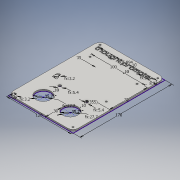
# Autodesk Inventor part: FrontPanel
Saved by Autodesk Inventor 2016 (Build 200138000, 138)
## iProperties
Created: 2015-09-18
Part Number: FrontPanel
Material: Generic
Document SubType Name: Modeling
Designer: Erin
Density: 1 g/cm^3
Appearance: Default
Author: Erin
Autodesk Inventor part; units mm, degrees
ref_plane "YZ Plane" through (0, 0, 0) normal (1, 0, 0) x (0, 1, 0)
ref_plane "XZ Plane" through (0, 0, 0) normal (0, 1, 0) x (-1, 0, 0)
ref_plane "XY Plane" through (0, 0, 0) normal (0, 0, 1) x (1, 0, 0)
sketch "Sketch1" plane through (0, 0, 0) normal (0, 0, 1) x (1, 0, 0)
  line L0 (-60, 85) -> (60, 85)
  line L1 (60, 85) -> (60, -85)
  line L2 (60, -85) -> (-60, -85)
  line L3 (-60, -85) -> (-60, 85)
  line L4 (-50, 56.6301) -> (50, 56.6301)
  line L5 (50, 56.6301) -> (50, -13.3699)
  line L6 (50, -13.3699) -> (-50, -13.3699)
  line L7 (-50, -13.3699) -> (-50, 56.6301)
  circle A0 centre (-25, -55) radius 13.85
  circle A1 centre (-25, -24.425) radius 2.7
  circle A2 centre (25, -24.425) radius 2.7
  line L8 (-25, 85) -> (-25, -85) construction
  line L9 (-60, -55) -> (60, -55) construction
  circle A3 centre (-25, -55) radius 17.875 construction
  line L10 (25, 85) -> (25, -85) construction
  circle A4 centre (25, -55) radius 13.85
  circle A5 centre (25, -55) radius 17.875 construction
  circle A6 centre (-53.4, -78.4) radius 1.6
  line L11 (-52.9471, 75) -> (52.9471, 75) construction
  line L12 (52.9471, 75) -> (52.9471, 66.6301) construction
  line L13 (52.9471, 66.6301) -> (-52.9471, 66.6301) construction
  line L14 (-52.9471, 66.6301) -> (-52.9471, 75) construction
  circle A7 centre (-43.4, -6.7699) radius 1.6
  line L15 (-50, 21.6301) -> (50, 21.6301) construction
  line L16 (0, 56.6301) -> (0, -13.3699) construction
  circle A8 centre (-43.4, 50.0301) radius 1.6
  circle A9 centre (43.4, -6.7699) radius 1.6
  circle A10 centre (43.4, 50.0301) radius 1.6
  line L17 (-60, 0) -> (60, 0) construction
  circle A11 centre (53.4, -78.4) radius 1.6
  circle A12 centre (-53.4, 78.4) radius 1.6
  circle A13 centre (53.4, 78.4) radius 1.6
  line L18 (-49.3691, 73.3171) -> (-49.3691, 72.0537)
  line L19 (-49.3691, 72.0537) -> (-50.4203, 72.0537)
  spline S0 degree 2 poles (-50.4203, 72.0537) (-50.6819, 72.0537) (-51.052, 71.6835) (-51.052, 71.422) knots 0 0 0 1 2 2 2
  line L20 (-51.052, 71.422) -> (-51.052, 70.3708)
  line L21 (-51.052, 70.3708) -> (-52.3154, 70.3708)
  line L22 (-52.3154, 70.3708) -> (-52.3154, 75)
  line L23 (-52.3154, 75) -> (-51.052, 75)
  line L24 (-51.052, 75) -> (-51.052, 73.9488)
  spline S1 degree 2 poles (-51.052, 73.9488) (-51.052, 73.6872) (-50.6819, 73.3171) (-50.4203, 73.3171) knots 0 0 0 1 2 2 2
  line L25 (-50.4203, 73.3171) -> (-49.3691, 73.3171)
  line L26 (-49.3691, 68.2634) -> (-49.3691, 67)
  line L27 (-49.3691, 67) -> (-50.4203, 67)
  spline S2 degree 2 poles (-50.4203, 67) (-50.8102, 67) (-51.506, 67.2961) (-52.0193, 67.8094) (-52.3154, 68.5052) (-52.3154, 68.8951) knots 0 0 0 1 2 3 4 4 4
  line L28 (-52.3154, 68.8951) -> (-52.3154, 69.9463)
  line L29 (-52.3154, 69.9463) -> (-51.052, 69.9463)
  line L30 (-51.052, 69.9463) -> (-51.052, 68.8951)
  spline S3 degree 2 poles (-51.052, 68.8951) (-51.052, 68.6336) (-50.6819, 68.2634) (-50.4203, 68.2634) knots 0 0 0 1 2 2 2
  line L31 (-50.4203, 68.2634) -> (-49.3691, 68.2634)
  line L32 (-45.1593, 73.3171) -> (-45.1593, 72.0537)
  line L33 (-45.1593, 72.0537) -> (-46.2105, 72.0537)
  spline S4 degree 2 poles (-46.2105, 72.0537) (-46.4721, 72.0537) (-46.8423, 71.6835) (-46.8423, 71.422) knots 0 0 0 1 2 2 2
  line L34 (-46.8423, 71.422) -> (-46.8423, 70.3708)
  line L35 (-46.8423, 70.3708) -> (-48.1057, 70.3708)
  line L36 (-48.1057, 70.3708) -> (-48.1057, 75)
  line L37 (-48.1057, 75) -> (-46.8423, 75)
  line L38 (-46.8423, 75) -> (-46.8423, 73.9488)
  spline S5 degree 2 poles (-46.8423, 73.9488) (-46.8423, 73.6872) (-46.4721, 73.3171) (-46.2105, 73.3171) knots 0 0 0 1 2 2 2
  line L39 (-46.2105, 73.3171) -> (-45.1593, 73.3171)
  line L40 (-44.7349, 72.0537) -> (-44.7349, 73.3171)
  line L41 (-44.7349, 73.3171) -> (-43.6837, 73.3171)
  spline S6 degree 2 poles (-43.6837, 73.3171) (-43.2938, 73.3171) (-42.598, 73.021) (-42.0847, 72.5077) (-41.7886, 71.8118) (-41.7886, 71.422) knots 0 0 0 1 2 3 4 4 4
  line L42 (-41.7886, 71.422) -> (-41.7886, 70.3708)
  line L43 (-41.7886, 70.3708) -> (-43.052, 70.3708)
  line L44 (-43.052, 70.3708) -> (-43.052, 71.422)
  spline S7 degree 2 poles (-43.052, 71.422) (-43.052, 71.6835) (-43.4123, 72.0537) (-43.6837, 72.0537) knots 0 0 0 1 2 2 2
  line L45 (-43.6837, 72.0537) -> (-44.7349, 72.0537)
  line L46 (-41.7886, 67) -> (-43.052, 67)
  line L47 (-43.052, 67) -> (-43.052, 69.9463)
  line L48 (-43.052, 69.9463) -> (-41.7886, 69.9463)
  line L49 (-41.7886, 69.9463) -> (-41.7886, 67)
  line L50 (-46.8423, 67) -> (-48.1057, 67)
  line L51 (-48.1057, 67) -> (-48.1057, 69.9463)
  line L52 (-48.1057, 69.9463) -> (-46.8423, 69.9463)
  line L53 (-46.8423, 69.9463) -> (-46.8423, 67)
  line L54 (-39.2617, 70.3708) -> (-40.5252, 70.3708)
  line L55 (-40.5252, 70.3708) -> (-40.5252, 71.422)
  spline S8 degree 2 poles (-40.5252, 71.422) (-40.5252, 71.8118) (-40.229, 72.5077) (-39.7158, 73.021) (-39.0199, 73.3171) (-38.63, 73.3171) knots 0 0 0 1 2 3 4 4 4
  line L56 (-38.63, 73.3171) -> (-37.5788, 73.3171)
  line L57 (-37.5788, 73.3171) -> (-37.5788, 72.0537)
  line L58 (-37.5788, 72.0537) -> (-38.63, 72.0537)
  spline S9 degree 2 poles (-38.63, 72.0537) (-38.8916, 72.0537) (-39.2617, 71.6835) (-39.2617, 71.422) knots 0 0 0 1 2 2 2
  line L59 (-39.2617, 71.422) -> (-39.2617, 70.3708)
  line L60 (-37.5788, 68.2634) -> (-37.5788, 67)
  line L61 (-37.5788, 67) -> (-38.63, 67)
  spline S10 degree 2 poles (-38.63, 67) (-39.0199, 67) (-39.7158, 67.2961) (-40.229, 67.8094) (-40.5252, 68.5052) (-40.5252, 68.8951) knots 0 0 0 1 2 3 4 4 4
  line L62 (-40.5252, 68.8951) -> (-40.5252, 69.9463)
  line L63 (-40.5252, 69.9463) -> (-39.2617, 69.9463)
  line L64 (-39.2617, 69.9463) -> (-39.2617, 68.8951)
  spline S11 degree 2 poles (-39.2617, 68.8951) (-39.2617, 68.6336) (-38.8916, 68.2634) (-38.63, 68.2634) knots 0 0 0 1 2 2 2
  line L65 (-38.63, 68.2634) -> (-37.5788, 68.2634)
  line L66 (-35.4715, 69.9463) -> (-34.2081, 69.9463)
  line L67 (-34.2081, 69.9463) -> (-34.2081, 68.8951)
  spline S12 degree 2 poles (-34.2081, 68.8951) (-34.2081, 68.5052) (-34.5042, 67.8094) (-35.0175, 67.2961) (-35.7133, 67) (-36.1032, 67) knots 0 0 0 1 2 3 4 4 4
  line L68 (-36.1032, 67) -> (-37.1544, 67)
  line L69 (-37.1544, 67) -> (-37.1544, 68.2634)
  line L70 (-37.1544, 68.2634) -> (-36.1032, 68.2634)
  spline S13 degree 2 poles (-36.1032, 68.2634) (-35.8318, 68.2634) (-35.4715, 68.6336) (-35.4715, 68.8951) knots 0 0 0 1 2 2 2
  line L71 (-35.4715, 68.8951) -> (-35.4715, 69.9463)
  line L72 (-37.1544, 72.0537) -> (-37.1544, 73.3171)
  line L73 (-37.1544, 73.3171) -> (-36.1032, 73.3171)
  spline S14 degree 2 poles (-36.1032, 73.3171) (-35.7133, 73.3171) (-35.0175, 73.021) (-34.5042, 72.5077) (-34.2081, 71.8118) (-34.2081, 71.422) knots 0 0 0 1 2 3 4 4 4
  line L74 (-34.2081, 71.422) -> (-34.2081, 70.3708)
  line L75 (-34.2081, 70.3708) -> (-35.4715, 70.3708)
  line L76 (-35.4715, 70.3708) -> (-35.4715, 71.422)
  spline S15 degree 2 poles (-35.4715, 71.422) (-35.4715, 71.6835) (-35.8318, 72.0537) (-36.1032, 72.0537) knots 0 0 0 1 2 2 2
  line L77 (-36.1032, 72.0537) -> (-37.1544, 72.0537)
  spline S16 degree 2 poles (-27.891, 68.8951) (-27.891, 68.6336) (-28.2513, 68.2634) (-28.5227, 68.2634) knots 0 0 0 1 2 2 2
  line L78 (-28.5227, 68.2634) -> (-29.5788, 68.2634)
  line L79 (-29.5788, 68.2634) -> (-29.5788, 67)
  line L80 (-29.5788, 67) -> (-28.5227, 67)
  spline S17 degree 2 poles (-28.5227, 67) (-28.1328, 67) (-27.4369, 67.2961) (-26.9237, 67.8094) (-26.6276, 68.5052) (-26.6276, 68.8951) knots 0 0 0 1 2 3 4 4 4
  line L81 (-26.6276, 68.8951) -> (-26.6276, 69.9463)
  line L82 (-26.6276, 69.9463) -> (-27.891, 69.9463)
  line L83 (-27.891, 69.9463) -> (-27.891, 68.8951)
  spline S18 degree 2 poles (-31.0495, 68.2634) (-31.3111, 68.2634) (-31.6812, 68.6336) (-31.6812, 68.8951) knots 0 0 0 1 2 2 2
  line L84 (-31.6812, 68.8951) -> (-31.6812, 69.9463)
  line L85 (-31.6812, 69.9463) -> (-32.9447, 69.9463)
  line L86 (-32.9447, 69.9463) -> (-32.9447, 68.8951)
  spline S19 degree 2 poles (-32.9447, 68.8951) (-32.9447, 68.5052) (-32.6485, 67.8094) (-32.1353, 67.2961) (-31.4394, 67) (-31.0495, 67) knots 0 0 0 1 2 3 4 4 4
  line L87 (-31.0495, 67) -> (-29.9983, 67)
  line L88 (-29.9983, 67) -> (-29.9983, 68.2634)
  line L89 (-29.9983, 68.2634) -> (-31.0495, 68.2634)
  line L90 (-32.9447, 73.3171) -> (-31.6812, 73.3171)
  line L91 (-31.6812, 73.3171) -> (-31.6812, 70.3708)
  line L92 (-31.6812, 70.3708) -> (-32.9447, 70.3708)
  line L93 (-32.9447, 70.3708) -> (-32.9447, 73.3171)
  line L94 (-27.891, 73.3171) -> (-26.6276, 73.3171)
  line L95 (-26.6276, 73.3171) -> (-26.6276, 70.3708)
  line L96 (-26.6276, 70.3708) -> (-27.891, 70.3708)
  line L97 (-27.891, 70.3708) -> (-27.891, 73.3171)
  line L98 (-20.73, 68.2634) -> (-20.73, 67)
  line L99 (-20.73, 67) -> (-23.469, 67)
  spline S20 degree 2 poles (-23.469, 67) (-23.8589, 67) (-24.5548, 67.2961) (-25.068, 67.8094) (-25.3641, 68.5052) (-25.3641, 68.8951) knots 0 0 0 1 2 3 4 4 4
  line L100 (-25.3641, 68.8951) -> (-25.3641, 69.9463)
  line L101 (-25.3641, 69.9463) -> (-24.1007, 69.9463)
  line L102 (-24.1007, 69.9463) -> (-24.1007, 68.8951)
  spline S21 degree 2 poles (-24.1007, 68.8951) (-24.1007, 68.6336) (-23.7306, 68.2634) (-23.469, 68.2634) knots 0 0 0 1 2 2 2
  line L103 (-23.469, 68.2634) -> (-20.73, 68.2634)
  line L104 (-20.3105, 69.9513) -> (-19.0471, 69.9513)
  line L105 (-19.0471, 69.9513) -> (-19.0471, 67.2122)
  spline S22 degree 2 poles (-19.0471, 67.2122) (-19.0471, 66.8223) (-19.3432, 66.1265) (-19.8564, 65.6132) (-20.5523, 65.3171) (-20.9422, 65.3171) knots 0 0 0 1 2 3 4 4 4
  line L106 (-20.9422, 65.3171) -> (-21.9934, 65.3171)
  line L107 (-21.9934, 65.3171) -> (-21.9934, 66.5805)
  line L108 (-21.9934, 66.5805) -> (-20.9422, 66.5805)
  spline S23 degree 2 poles (-20.9422, 66.5805) (-20.6708, 66.5805) (-20.3105, 66.9506) (-20.3105, 67.2122) knots 0 0 0 1 2 2 2
  line L109 (-20.3105, 67.2122) -> (-20.3105, 69.9513)
  line L110 (-24.1007, 70.3708) -> (-25.3641, 70.3708)
  line L111 (-25.3641, 70.3708) -> (-25.3641, 71.422)
  spline S24 degree 2 poles (-25.3641, 71.422) (-25.3641, 71.8118) (-25.068, 72.5077) (-24.5548, 73.021) (-23.8589, 73.3171) (-23.469, 73.3171) knots 0 0 0 1 2 3 4 4 4
  line L112 (-23.469, 73.3171) -> (-22.4178, 73.3171)
  line L113 (-22.4178, 73.3171) -> (-22.4178, 72.0537)
  line L114 (-22.4178, 72.0537) -> (-23.469, 72.0537)
  spline S25 degree 2 poles (-23.469, 72.0537) (-23.7306, 72.0537) (-24.1007, 71.6835) (-24.1007, 71.422) knots 0 0 0 1 2 2 2
  line L115 (-24.1007, 71.422) -> (-24.1007, 70.3708)
  line L116 (-21.9934, 72.0537) -> (-21.9934, 73.3171)
  line L117 (-21.9934, 73.3171) -> (-20.9422, 73.3171)
  spline S26 degree 2 poles (-20.9422, 73.3171) (-20.5523, 73.3171) (-19.8564, 73.021) (-19.3432, 72.5077) (-19.0471, 71.8118) (-19.0471, 71.422) knots 0 0 0 1 2 3 4 4 4
  line L118 (-19.0471, 71.422) -> (-19.0471, 70.3708)
  line L119 (-19.0471, 70.3708) -> (-20.3105, 70.3708)
  line L120 (-20.3105, 70.3708) -> (-20.3105, 71.422)
  spline S27 degree 2 poles (-20.3105, 71.422) (-20.3105, 71.6835) (-20.6708, 72.0537) (-20.9422, 72.0537) knots 0 0 0 1 2 2 2
  line L121 (-20.9422, 72.0537) -> (-21.9934, 72.0537)
  line L122 (-22.4178, 66.5805) -> (-22.4178, 65.3171)
  line L123 (-22.4178, 65.3171) -> (-25.3641, 65.3171)
  line L124 (-25.3641, 65.3171) -> (-25.3641, 66.5805)
  line L125 (-25.3641, 66.5805) -> (-22.4178, 66.5805)
  line L126 (-14.8373, 73.3171) -> (-14.8373, 72.0537)
  line L127 (-14.8373, 72.0537) -> (-15.8885, 72.0537)
  spline S28 degree 2 poles (-15.8885, 72.0537) (-16.1501, 72.0537) (-16.5202, 71.6835) (-16.5202, 71.422) knots 0 0 0 1 2 2 2
  line L128 (-16.5202, 71.422) -> (-16.5202, 70.3708)
  line L129 (-16.5202, 70.3708) -> (-17.7836, 70.3708)
  line L130 (-17.7836, 70.3708) -> (-17.7836, 75)
  line L131 (-17.7836, 75) -> (-16.5202, 75)
  line L132 (-16.5202, 75) -> (-16.5202, 73.9488)
  spline S29 degree 2 poles (-16.5202, 73.9488) (-16.5202, 73.6872) (-16.1501, 73.3171) (-15.8885, 73.3171) knots 0 0 0 1 2 2 2
  line L133 (-15.8885, 73.3171) -> (-14.8373, 73.3171)
  line L134 (-14.4129, 72.0537) -> (-14.4129, 73.3171)
  line L135 (-14.4129, 73.3171) -> (-13.3617, 73.3171)
  spline S30 degree 2 poles (-13.3617, 73.3171) (-12.9718, 73.3171) (-12.2759, 73.021) (-11.7627, 72.5077) (-11.4666, 71.8118) (-11.4666, 71.422) knots 0 0 0 1 2 3 4 4 4
  line L136 (-11.4666, 71.422) -> (-11.4666, 70.3708)
  line L137 (-11.4666, 70.3708) -> (-12.73, 70.3708)
  line L138 (-12.73, 70.3708) -> (-12.73, 71.422)
  spline S31 degree 2 poles (-12.73, 71.422) (-12.73, 71.6835) (-13.0902, 72.0537) (-13.3617, 72.0537) knots 0 0 0 1 2 2 2
  line L139 (-13.3617, 72.0537) -> (-14.4129, 72.0537)
  line L140 (-11.4666, 67) -> (-12.73, 67)
  line L141 (-12.73, 67) -> (-12.73, 69.9463)
  line L142 (-12.73, 69.9463) -> (-11.4666, 69.9463)
  line L143 (-11.4666, 69.9463) -> (-11.4666, 67)
  line L144 (-16.5202, 67) -> (-17.7836, 67)
  line L145 (-17.7836, 67) -> (-17.7836, 69.9463)
  line L146 (-17.7836, 69.9463) -> (-16.5202, 69.9463)
  line L147 (-16.5202, 69.9463) -> (-16.5202, 67)
  line L148 (-7.2568, 73.3171) -> (-7.2568, 72.0537)
  line L149 (-7.2568, 72.0537) -> (-8.308, 72.0537)
  spline S32 degree 2 poles (-8.308, 72.0537) (-8.5696, 72.0537) (-8.9397, 71.6835) (-8.9397, 71.422) knots 0 0 0 1 2 2 2
  line L150 (-8.9397, 71.422) -> (-8.9397, 70.3708)
  line L151 (-8.9397, 70.3708) -> (-10.2031, 70.3708)
  line L152 (-10.2031, 70.3708) -> (-10.2031, 75)
  line L153 (-10.2031, 75) -> (-8.9397, 75)
  line L154 (-8.9397, 75) -> (-8.9397, 73.9488)
  spline S33 degree 2 poles (-8.9397, 73.9488) (-8.9397, 73.6872) (-8.5696, 73.3171) (-8.308, 73.3171) knots 0 0 0 1 2 2 2
  line L155 (-8.308, 73.3171) -> (-7.2568, 73.3171)
  line L156 (-7.2568, 68.2634) -> (-7.2568, 67)
  line L157 (-7.2568, 67) -> (-8.308, 67)
  spline S34 degree 2 poles (-8.308, 67) (-8.6979, 67) (-9.3938, 67.2961) (-9.907, 67.8094) (-10.2031, 68.5052) (-10.2031, 68.8951) knots 0 0 0 1 2 3 4 4 4
  line L158 (-10.2031, 68.8951) -> (-10.2031, 69.9463)
  line L159 (-10.2031, 69.9463) -> (-8.9397, 69.9463)
  line L160 (-8.9397, 69.9463) -> (-8.9397, 68.8951)
  spline S35 degree 2 poles (-8.9397, 68.8951) (-8.9397, 68.6336) (-8.5696, 68.2634) (-8.308, 68.2634) knots 0 0 0 1 2 2 2
  line L161 (-8.308, 68.2634) -> (-7.2568, 68.2634)
  spline S36 degree 2 poles (-1.1519, 67) (-1.4135, 67) (-1.7836, 66.6299) (-1.7836, 66.3683) knots 0 0 0 1 2 2 2
  line L162 (-1.7836, 66.3683) -> (-1.7836, 65.3171)
  line L163 (-1.7836, 65.3171) -> (-3.0471, 65.3171)
  line L164 (-3.0471, 65.3171) -> (-3.0471, 69.9463)
  line L165 (-3.0471, 69.9463) -> (-1.7836, 69.9463)
  line L166 (-1.7836, 69.9463) -> (-1.7836, 68.8951)
  spline S37 degree 2 poles (-1.7836, 68.8951) (-1.7836, 68.6336) (-1.4135, 68.2634) (-1.1519, 68.2634) knots 0 0 0 1 2 2 2
  line L167 (-1.1519, 68.2634) -> (-0.1007, 68.2634)
  line L168 (-0.1007, 68.2634) -> (-0.1007, 67)
  line L169 (-0.1007, 67) -> (-1.1519, 67)
  spline S38 degree 2 poles (-1.1519, 72.0537) (-1.4135, 72.0537) (-1.7836, 71.6835) (-1.7836, 71.422) knots 0 0 0 1 2 2 2
  line L170 (-1.7836, 71.422) -> (-1.7836, 70.3708)
  line L171 (-1.7836, 70.3708) -> (-3.0471, 70.3708)
  line L172 (-3.0471, 70.3708) -> (-3.0471, 71.422)
  spline S39 degree 2 poles (-3.0471, 71.422) (-3.0471, 71.8118) (-2.7509, 72.5077) (-2.2377, 73.021) (-1.5418, 73.3171) (-1.1519, 73.3171) knots 0 0 0 1 2 3 4 4 4
  line L173 (-1.1519, 73.3171) -> (-0.1007, 73.3171)
  line L174 (-0.1007, 73.3171) -> (-0.1007, 72.0537)
  line L175 (-0.1007, 72.0537) -> (-1.1519, 72.0537)
  spline S40 degree 2 poles (2.0066, 71.422) (2.0066, 71.6835) (1.6463, 72.0537) (1.3749, 72.0537) knots 0 0 0 1 2 2 2
  line L176 (1.3749, 72.0537) -> (0.3237, 72.0537)
  line L177 (0.3237, 72.0537) -> (0.3237, 73.3171)
  line L178 (0.3237, 73.3171) -> (1.3749, 73.3171)
  spline S41 degree 2 poles (1.3749, 73.3171) (1.7648, 73.3171) (2.4607, 73.021) (2.9739, 72.5077) (3.27, 71.8118) (3.27, 71.422) knots 0 0 0 1 2 3 4 4 4
  line L179 (3.27, 71.422) -> (3.27, 70.3708)
  line L180 (3.27, 70.3708) -> (2.0066, 70.3708)
  line L181 (2.0066, 70.3708) -> (2.0066, 71.422)
  spline S42 degree 2 poles (1.3749, 68.2634) (1.6463, 68.2634) (2.0066, 68.6336) (2.0066, 68.8951) knots 0 0 0 1 2 2 2
  line L182 (2.0066, 68.8951) -> (2.0066, 69.9463)
  line L183 (2.0066, 69.9463) -> (3.27, 69.9463)
  line L184 (3.27, 69.9463) -> (3.27, 68.8951)
  spline S43 degree 2 poles (3.27, 68.8951) (3.27, 68.5052) (2.9739, 67.8094) (2.4607, 67.2961) (1.7648, 67) (1.3749, 67) knots 0 0 0 1 2 3 4 4 4
  line L185 (1.3749, 67) -> (0.3237, 67)
  line L186 (0.3237, 67) -> (0.3237, 68.2634)
  line L187 (0.3237, 68.2634) -> (1.3749, 68.2634)
  spline S44 degree 2 poles (6.4286, 72.0537) (6.167, 72.0537) (5.7969, 71.6835) (5.7969, 71.422) knots 0 0 0 1 2 2 2
  line L188 (5.7969, 71.422) -> (5.7969, 70.3708)
  line L189 (5.7969, 70.3708) -> (4.5334, 70.3708)
  line L190 (4.5334, 70.3708) -> (4.5334, 71.422)
  spline S45 degree 2 poles (4.5334, 71.422) (4.5334, 71.8118) (4.8296, 72.5077) (5.3428, 73.021) (6.0387, 73.3171) (6.4286, 73.3171) knots 0 0 0 1 2 3 4 4 4
  line L191 (6.4286, 73.3171) -> (9.1676, 73.3171)
  line L192 (9.1676, 73.3171) -> (9.1676, 72.0537)
  line L193 (9.1676, 72.0537) -> (6.4286, 72.0537)
  line L194 (5.7969, 67) -> (4.5334, 67)
  line L195 (4.5334, 67) -> (4.5334, 69.9463)
  line L196 (4.5334, 69.9463) -> (5.7969, 69.9463)
  line L197 (5.7969, 69.9463) -> (5.7969, 67)
  line L198 (11.6895, 70.3708) -> (10.4261, 70.3708)
  line L199 (10.4261, 70.3708) -> (10.4261, 71.422)
  spline S46 degree 2 poles (10.4261, 71.422) (10.4261, 71.8118) (10.7222, 72.5077) (11.2355, 73.021) (11.9313, 73.3171) (12.3212, 73.3171) knots 0 0 0 1 2 3 4 4 4
  line L200 (12.3212, 73.3171) -> (13.3724, 73.3171)
  line L201 (13.3724, 73.3171) -> (13.3724, 72.0537)
  line L202 (13.3724, 72.0537) -> (12.3212, 72.0537)
  spline S47 degree 2 poles (12.3212, 72.0537) (12.0597, 72.0537) (11.6895, 71.6835) (11.6895, 71.422) knots 0 0 0 1 2 2 2
  line L203 (11.6895, 71.422) -> (11.6895, 70.3708)
  line L204 (13.3724, 68.2634) -> (13.3724, 67)
  line L205 (13.3724, 67) -> (12.3212, 67)
  spline S48 degree 2 poles (12.3212, 67) (11.9313, 67) (11.2355, 67.2961) (10.7222, 67.8094) (10.4261, 68.5052) (10.4261, 68.8951) knots 0 0 0 1 2 3 4 4 4
  line L206 (10.4261, 68.8951) -> (10.4261, 69.9463)
  line L207 (10.4261, 69.9463) -> (11.6895, 69.9463)
  line L208 (11.6895, 69.9463) -> (11.6895, 68.8951)
  spline S49 degree 2 poles (11.6895, 68.8951) (11.6895, 68.6336) (12.0597, 68.2634) (12.3212, 68.2634) knots 0 0 0 1 2 2 2
  line L209 (12.3212, 68.2634) -> (13.3724, 68.2634)
  line L210 (13.7969, 72.0537) -> (13.7969, 73.3171)
  line L211 (13.7969, 73.3171) -> (14.8481, 73.3171)
  spline S50 degree 2 poles (14.8481, 73.3171) (15.2379, 73.3171) (15.9338, 73.021) (16.4471, 72.5077) (16.7432, 71.8118) (16.7432, 71.422) knots 0 0 0 1 2 3 4 4 4
  line L212 (16.7432, 71.422) -> (16.7432, 70.3708)
  line L213 (16.7432, 70.3708) -> (15.4798, 70.3708)
  line L214 (15.4798, 70.3708) -> (15.4798, 71.422)
  spline S51 degree 2 poles (15.4798, 71.422) (15.4798, 71.6835) (15.1195, 72.0537) (14.8481, 72.0537) knots 0 0 0 1 2 2 2
  line L215 (14.8481, 72.0537) -> (13.7969, 72.0537)
  line L216 (15.4798, 69.9463) -> (16.7432, 69.9463)
  line L217 (16.7432, 69.9463) -> (16.7432, 68.8951)
  spline S52 degree 2 poles (16.7432, 68.8951) (16.7432, 68.5052) (16.4471, 67.8094) (15.9338, 67.2961) (15.2379, 67) (14.8481, 67) knots 0 0 0 1 2 3 4 4 4
  line L218 (14.8481, 67) -> (13.7969, 67)
  line L219 (13.7969, 67) -> (13.7969, 68.2634)
  line L220 (13.7969, 68.2634) -> (14.8481, 68.2634)
  spline S53 degree 2 poles (14.8481, 68.2634) (15.1195, 68.2634) (15.4798, 68.6336) (15.4798, 68.8951) knots 0 0 0 1 2 2 2
  line L221 (15.4798, 68.8951) -> (15.4798, 69.9463)
  spline S54 degree 2 poles (20.7457, 72.0537) (21.0171, 72.0537) (21.3774, 71.6835) (21.3774, 71.422) knots 0 0 0 1 2 2 2
  line L222 (21.3774, 71.422) -> (21.3774, 70.3708)
  line L223 (21.3774, 70.3708) -> (22.6408, 70.3708)
  line L224 (22.6408, 70.3708) -> (22.6408, 71.422)
  spline S55 degree 2 poles (22.6408, 71.422) (22.6408, 71.8118) (22.3447, 72.5077) (21.8314, 73.021) (21.1355, 73.3171) (20.7457, 73.3171) knots 0 0 0 1 2 3 4 4 4
  line L225 (20.7457, 73.3171) -> (19.6945, 73.3171)
  line L226 (19.6945, 73.3171) -> (19.6945, 72.0537)
  line L227 (19.6945, 72.0537) -> (20.7457, 72.0537)
  spline S56 degree 2 poles (24.1115, 72.0537) (24.3879, 72.0537) (24.7432, 71.6835) (24.7432, 71.422) knots 0 0 0 1 2 2 2
  line L228 (24.7432, 71.422) -> (24.7432, 70.3708)
  line L229 (24.7432, 70.3708) -> (26.0066, 70.3708)
  line L230 (26.0066, 70.3708) -> (26.0066, 71.422)
  spline S57 degree 2 poles (26.0066, 71.422) (26.0066, 71.8118) (25.7105, 72.5077) (25.1972, 73.021) (24.5014, 73.3171) (24.1115, 73.3171) knots 0 0 0 1 2 3 4 4 4
  line L231 (24.1115, 73.3171) -> (23.0603, 73.3171)
  line L232 (23.0603, 73.3171) -> (23.0603, 72.0537)
  line L233 (23.0603, 72.0537) -> (24.1115, 72.0537)
  line L234 (26.0066, 67) -> (24.7432, 67)
  line L235 (24.7432, 67) -> (24.7432, 69.9463)
  line L236 (24.7432, 69.9463) -> (26.0066, 69.9463)
  line L237 (26.0066, 69.9463) -> (26.0066, 67)
  line L238 (22.6408, 67) -> (21.3774, 67)
  line L239 (21.3774, 67) -> (21.3774, 69.9463)
  line L240 (21.3774, 69.9463) -> (22.6408, 69.9463)
  line L241 (22.6408, 69.9463) -> (22.6408, 67)
  line L242 (19.27, 70.3708) -> (18.0066, 70.3708)
  line L243 (18.0066, 70.3708) -> (18.0066, 73.3171)
  line L244 (18.0066, 73.3171) -> (19.27, 73.3171)
  line L245 (19.27, 73.3171) -> (19.27, 70.3708)
  line L246 (19.27, 67) -> (18.0066, 67)
  line L247 (18.0066, 67) -> (18.0066, 69.9463)
  line L248 (18.0066, 69.9463) -> (19.27, 69.9463)
  line L249 (19.27, 69.9463) -> (19.27, 67)
  spline S58 degree 2 poles (29.1652, 67) (28.9036, 67) (28.5334, 66.6299) (28.5334, 66.3683) knots 0 0 0 1 2 2 2
  line L250 (28.5334, 66.3683) -> (28.5334, 65.3171)
  line L251 (28.5334, 65.3171) -> (27.27, 65.3171)
  line L252 (27.27, 65.3171) -> (27.27, 69.9463)
  line L253 (27.27, 69.9463) -> (28.5334, 69.9463)
  line L254 (28.5334, 69.9463) -> (28.5334, 68.8951)
  spline S59 degree 2 poles (28.5334, 68.8951) (28.5334, 68.6336) (28.9036, 68.2634) (29.1652, 68.2634) knots 0 0 0 1 2 2 2
  line L255 (29.1652, 68.2634) -> (30.2164, 68.2634)
  line L256 (30.2164, 68.2634) -> (30.2164, 67)
  line L257 (30.2164, 67) -> (29.1652, 67)
  spline S60 degree 2 poles (29.1652, 72.0537) (28.9036, 72.0537) (28.5334, 71.6835) (28.5334, 71.422) knots 0 0 0 1 2 2 2
  line L258 (28.5334, 71.422) -> (28.5334, 70.3708)
  line L259 (28.5334, 70.3708) -> (27.27, 70.3708)
  line L260 (27.27, 70.3708) -> (27.27, 71.422)
  spline S61 degree 2 poles (27.27, 71.422) (27.27, 71.8118) (27.5661, 72.5077) (28.0794, 73.021) (28.7753, 73.3171) (29.1652, 73.3171) knots 0 0 0 1 2 3 4 4 4
  line L261 (29.1652, 73.3171) -> (30.2164, 73.3171)
  line L262 (30.2164, 73.3171) -> (30.2164, 72.0537)
  line L263 (30.2164, 72.0537) -> (29.1652, 72.0537)
  spline S62 degree 2 poles (32.3237, 71.422) (32.3237, 71.6835) (31.9634, 72.0537) (31.692, 72.0537) knots 0 0 0 1 2 2 2
  line L264 (31.692, 72.0537) -> (30.6408, 72.0537)
  line L265 (30.6408, 72.0537) -> (30.6408, 73.3171)
  line L266 (30.6408, 73.3171) -> (31.692, 73.3171)
  spline S63 degree 2 poles (31.692, 73.3171) (32.0819, 73.3171) (32.7777, 73.021) (33.291, 72.5077) (33.5871, 71.8118) (33.5871, 71.422) knots 0 0 0 1 2 3 4 4 4
  line L267 (33.5871, 71.422) -> (33.5871, 70.3708)
  line L268 (33.5871, 70.3708) -> (32.3237, 70.3708)
  line L269 (32.3237, 70.3708) -> (32.3237, 71.422)
  spline S64 degree 2 poles (31.692, 68.2634) (31.9634, 68.2634) (32.3237, 68.6336) (32.3237, 68.8951) knots 0 0 0 1 2 2 2
  line L270 (32.3237, 68.8951) -> (32.3237, 69.9463)
  line L271 (32.3237, 69.9463) -> (33.5871, 69.9463)
  line L272 (33.5871, 69.9463) -> (33.5871, 68.8951)
  spline S65 degree 2 poles (33.5871, 68.8951) (33.5871, 68.5052) (33.291, 67.8094) (32.7777, 67.2961) (32.0819, 67) (31.692, 67) knots 0 0 0 1 2 3 4 4 4
  line L273 (31.692, 67) -> (30.6408, 67)
  line L274 (30.6408, 67) -> (30.6408, 68.2634)
  line L275 (30.6408, 68.2634) -> (31.692, 68.2634)
  line L276 (37.7969, 73.3171) -> (37.7969, 72.0537)
  line L277 (37.7969, 72.0537) -> (36.7457, 72.0537)
  spline S66 degree 2 poles (36.7457, 72.0537) (36.4841, 72.0537) (36.114, 71.6835) (36.114, 71.422) knots 0 0 0 1 2 2 2
  line L278 (36.114, 71.422) -> (36.114, 70.3708)
  line L279 (36.114, 70.3708) -> (34.8505, 70.3708)
  line L280 (34.8505, 70.3708) -> (34.8505, 75)
  line L281 (34.8505, 75) -> (36.114, 75)
  line L282 (36.114, 75) -> (36.114, 73.9488)
  spline S67 degree 2 poles (36.114, 73.9488) (36.114, 73.6872) (36.4841, 73.3171) (36.7457, 73.3171) knots 0 0 0 1 2 2 2
  line L283 (36.7457, 73.3171) -> (37.7969, 73.3171)
  line L284 (37.7969, 68.2634) -> (37.7969, 67)
  line L285 (37.7969, 67) -> (36.7457, 67)
  spline S68 degree 2 poles (36.7457, 67) (36.3558, 67) (35.6599, 67.2961) (35.1466, 67.8094) (34.8505, 68.5052) (34.8505, 68.8951) knots 0 0 0 1 2 3 4 4 4
  line L286 (34.8505, 68.8951) -> (34.8505, 69.9463)
  line L287 (34.8505, 69.9463) -> (36.114, 69.9463)
  line L288 (36.114, 69.9463) -> (36.114, 68.8951)
  spline S69 degree 2 poles (36.114, 68.8951) (36.114, 68.6336) (36.4841, 68.2634) (36.7457, 68.2634) knots 0 0 0 1 2 2 2
  line L289 (36.7457, 68.2634) -> (37.7969, 68.2634)
  spline S70 degree 2 poles (44.114, 71.422) (44.114, 71.6835) (43.7537, 72.0537) (43.4822, 72.0537) knots 0 0 0 1 2 2 2
  line L290 (43.4822, 72.0537) -> (42.431, 72.0537)
  line L291 (42.431, 72.0537) -> (42.431, 73.3171)
  line L292 (42.431, 73.3171) -> (43.4822, 73.3171)
  spline S71 degree 2 poles (43.4822, 73.3171) (43.8721, 73.3171) (44.568, 73.021) (45.0813, 72.5077) (45.3774, 71.8118) (45.3774, 71.422) knots 0 0 0 1 2 3 4 4 4
  line L293 (45.3774, 71.422) -> (45.3774, 70.578)
  spline S72 degree 2 poles (45.3774, 70.578) (45.3774, 70.1882) (45.0813, 69.4923) (44.568, 68.979) (43.8721, 68.6829) (43.4822, 68.6829) knots 0 0 0 1 2 3 4 4 4
  line L294 (43.4822, 68.6829) -> (42.431, 68.6829)
  line L295 (42.431, 68.6829) -> (42.431, 69.9463)
  line L296 (42.431, 69.9463) -> (43.4822, 69.9463)
  spline S73 degree 2 poles (43.4822, 69.9463) (43.7537, 69.9463) (44.114, 70.3165) (44.114, 70.578) knots 0 0 0 1 2 2 2
  line L297 (44.114, 70.578) -> (44.114, 71.422)
  line L298 (40.3237, 70.3708) -> (39.0603, 70.3708)
  line L299 (39.0603, 70.3708) -> (39.0603, 71.422)
  spline S74 degree 2 poles (39.0603, 71.422) (39.0603, 71.8118) (39.3564, 72.5077) (39.8697, 73.021) (40.5655, 73.3171) (40.9554, 73.3171) knots 0 0 0 1 2 3 4 4 4
  line L300 (40.9554, 73.3171) -> (42.0066, 73.3171)
  line L301 (42.0066, 73.3171) -> (42.0066, 72.0537)
  line L302 (42.0066, 72.0537) -> (40.9554, 72.0537)
  spline S75 degree 2 poles (40.9554, 72.0537) (40.6938, 72.0537) (40.3237, 71.6835) (40.3237, 71.422) knots 0 0 0 1 2 2 2
  line L303 (40.3237, 71.422) -> (40.3237, 70.3708)
  line L304 (42.0066, 68.2634) -> (42.0066, 67)
  line L305 (42.0066, 67) -> (40.9554, 67)
  spline S76 degree 2 poles (40.9554, 67) (40.5655, 67) (39.8697, 67.2961) (39.3564, 67.8094) (39.0603, 68.5052) (39.0603, 68.8951) knots 0 0 0 1 2 3 4 4 4
  line L306 (39.0603, 68.8951) -> (39.0603, 69.9463)
  line L307 (39.0603, 69.9463) -> (40.3237, 69.9463)
  line L308 (40.3237, 69.9463) -> (40.3237, 68.8951)
  spline S77 degree 2 poles (40.3237, 68.8951) (40.3237, 68.6336) (40.6938, 68.2634) (40.9554, 68.2634) knots 0 0 0 1 2 2 2
  line L309 (40.9554, 68.2634) -> (42.0066, 68.2634)
  line L310 (45.3774, 68.2634) -> (45.3774, 67)
  line L311 (45.3774, 67) -> (42.431, 67)
  line L312 (42.431, 67) -> (42.431, 68.2634)
  line L313 (42.431, 68.2634) -> (45.3774, 68.2634)
  spline S78 degree 2 poles (48.5359, 72.0537) (48.2743, 72.0537) (47.9042, 71.6835) (47.9042, 71.422) knots 0 0 0 1 2 2 2
  line L314 (47.9042, 71.422) -> (47.9042, 70.3708)
  line L315 (47.9042, 70.3708) -> (46.6408, 70.3708)
  line L316 (46.6408, 70.3708) -> (46.6408, 71.422)
  spline S79 degree 2 poles (46.6408, 71.422) (46.6408, 71.8118) (46.9369, 72.5077) (47.4502, 73.021) (48.146, 73.3171) (48.5359, 73.3171) knots 0 0 0 1 2 3 4 4 4
  line L317 (48.5359, 73.3171) -> (51.275, 73.3171)
  line L318 (51.275, 73.3171) -> (51.275, 72.0537)
  line L319 (51.275, 72.0537) -> (48.5359, 72.0537)
  line L320 (47.9042, 67) -> (46.6408, 67)
  line L321 (46.6408, 67) -> (46.6408, 69.9463)
  line L322 (46.6408, 69.9463) -> (47.9042, 69.9463)
  line L323 (47.9042, 69.9463) -> (47.9042, 67)
  point P0 (0, 0)
  point P1 (0, 85)
  point P2 (0, 75)
  dimension "d0" = 120
  dimension "d1" = 170
  dimension "d2" = 27.7
  dimension "d4" = 5.4
  dimension "d5" = 5.4
  dimension "d10" = 35
  dimension "d11" = 30
  dimension "d12" = 35.75
  dimension "d13" = 10
  dimension "d14" = 35
  dimension "d15" = 27.7
  dimension "d16" = 35.75
  dimension "d17" = 10
  dimension "d18" = 3.2
  dimension "d19" = 5
  dimension "d21" = 5
  dimension "d22" = 10
  dimension "d23" = 10
  dimension "d24" = 100
  dimension "d25" = 70
  dimension "d26" = 8.3699
  dimension "d27" = 8.3551
  dimension "d28" = 3.2
  dimension "d29" = 5
  dimension "d30" = 5
  dimension "d31" = 105.8942
  constraints: 28 end point, 14 centre point, 12 point on line, 8 midpoint, 6 symmetric about line, 4 parallel, 4 perpendicular, 3 horizontal, 3 vertical alignment, 2 coincident, 1 horizontal alignment, 1 vertical, 8 other
  measures "d0" distance of L1.end L2.end
  measures "d1" distance of L0.end L1.end
  measures "d2" diameter of A0
  measures "d4" diameter of A1
  measures "d5" diameter of A2
  measures "d10" distance between parallel lines of L3 L8
  measures "d11" distance between parallel lines of L9 L2
  measures "d12" diameter of A3
  measures "d14" distance between parallel lines of L10 L1
  measures "d15" diameter of A4
  measures "d16" diameter of A5
  measures "d18" diameter of A6
  measures "d19" distance edge to line of A6 L2
  measures "d21" distance edge to line of A6 L3
  measures "d22" distance between parallel lines of L13 L4
  measures "d23" distance between parallel lines of L0 L11
  measures "d24" distance of L4.start L4.end
  measures "d25" distance of L4.end L5.end
  measures "d26" distance of L11.end L12.end
  measures "d27" distance edge to line of A2 L6
  measures "d28" diameter of A7
  measures "d29" distance edge to line of A7 L6
  measures "d30" distance edge to line of A7 L7
  measures "d31" distance of L11.start L11.end
extrude "Extrusion1" add sketch "Sketch1" along normal blind 3 contours L0 L1 L2 L3 | L4 L5 L6 L7 | L18 L19 S0 L20 L21 L22 L23 L24 S1 L25 | L26 L27 S2 L28 L29 L30 S3 L31 | L32 L33 S4 L34 L35 L36 L37 L38 S5 L39 | L40 L41 S6 L42 L43 L44 S7 L45 | L46 L47 L48 L49 | L50 L51 L52 L53 | L54 L55 S8 L56 L57 L58 S9 L59 | L60 L61 S10 L62 L63 L64 S11 L65 | L66 L67 S12 L68 L69 L70 S13 L71 | L72 L73 S14 L74 L75 L76 S15 L77 | L83 L82 L81 S17 L80 L79 L78 S16 | L89 L88 L87 S19 L86 L85 L84 S18 | L90 L91 L92 L93 | L94 L95 L96 L97 | L98 L99 S20 L100 L101 L102 S21 L103 | L104 L105 S22 L106 L107 L108 S23 L109 | L110 L111 S24 L112 L113 L114 S25 L115 | L116 L117 S26 L118 L119 L120 S27 L121 | L122 L123 L124 L125 | L126 L127 S28 L128 L129 L130 L131 L132 S29 L133 | L134 L135 S30 L136 L137 L138 S31 L139 | L140 L141 L142 L143 | L144 L145 L146 L147 | L148 L149 S32 L150 L151 L152 L153 L154 S33 L155 | L156 L157 S34 L158 L159 L160 S35 L161 | S36 L162 L163 L164 L165 L166 S37 L167 L168 L169 | S38 L170 L171 L172 S39 L173 L174 L175 | S40 L176 L177 L178 S41 L179 L180 L181 | S42 L182 L183 L184 S43 L185 L186 L187 | S44 L188 L189 L190 S45 L191 L192 L193 | L194 L195 L196 L197 | L198 L199 S46 L200 L201 L202 S47 L203 | L204 L205 S48 L206 L207 L208 S49 L209 | L210 L211 S50 L212 L213 L214 S51 L215 | L216 L217 S52 L218 L219 L220 S53 L221 | L227 L226 L225 S55 L224 L223 L222 S54 | L233 L232 L231 S57 L230 L229 L228 S56 | L234 L235 L236 L237 | L238 L239 L240 L241 | L242 L243 L244 L245 | L246 L247 L248 L249 | S58 L250 L251 L252 L253 L254 S59 L255 L256 L257 | S60 L258 L259 L260 S61 L261 L262 L263 | S62 L264 L265 L266 S63 L267 L268 L269 | S64 L270 L271 L272 S65 L273 L274 L275 | L276 L277 S66 L278 L279 L280 L281 L282 S67 L283 | L284 L285 S68 L286 L287 L288 S69 L289 | S70 L290 L291 L292 S71 L293 S72 L294 L295 L296 S73 L297 | L298 L299 S74 L300 L301 L302 S75 L303 | L304 L305 S76 L306 L307 L308 S77 L309 | L310 L311 L312 L313 | S78 L314 L315 L316 S79 L317 L318 L319 | L320 L321 L322 L323
fillet "Fillet1" radius 10 4 edges at (-60, -85, 1.5) (60, -85, 1.5) (60, 85, 1.5) (-60, 85, 1.5)
extrude "Extrusion2" cut sketch "Sketch1" along normal blind 4 contours L18 L19 S0 L20 L21 L22 L23 L24 S1 L25 | L26 L27 S2 L28 L29 L30 S3 L31 | L32 L33 S4 L34 L35 L36 L37 L38 S5 L39 | L40 L41 S6 L42 L43 L44 S7 L45 | L46 L47 L48 L49 | L50 L51 L52 L53 | L54 L55 S8 L56 L57 L58 S9 L59 | L60 L61 S10 L62 L63 L64 S11 L65 | L66 L67 S12 L68 L69 L70 S13 L71 | L72 L73 S14 L74 L75 L76 S15 L77 | L83 L82 L81 S17 L80 L79 L78 S16 | L89 L88 L87 S19 L86 L85 L84 S18 | L90 L91 L92 L93 | L94 L95 L96 L97 | L98 L99 S20 L100 L101 L102 S21 L103 | L104 L105 S22 L106 L107 L108 S23 L109 | L110 L111 S24 L112 L113 L114 S25 L115 | L116 L117 S26 L118 L119 L120 S27 L121 | L122 L123 L124 L125 | L126 L127 S28 L128 L129 L130 L131 L132 S29 L133 | L134 L135 S30 L136 L137 L138 S31 L139 | L140 L141 L142 L143 | L144 L145 L146 L147 | L148 L149 S32 L150 L151 L152 L153 L154 S33 L155 | L156 L157 S34 L158 L159 L160 S35 L161 | S36 L162 L163 L164 L165 L166 S37 L167 L168 L169 | S38 L170 L171 L172 S39 L173 L174 L175 | S40 L176 L177 L178 S41 L179 L180 L181 | S42 L182 L183 L184 S43 L185 L186 L187 | S44 L188 L189 L190 S45 L191 L192 L193 | L194 L195 L196 L197 | L198 L199 S46 L200 L201 L202 S47 L203 | L204 L205 S48 L206 L207 L208 S49 L209 | L210 L211 S50 L212 L213 L214 S51 L215 | L216 L217 S52 L218 L219 L220 S53 L221 | L227 L226 L225 S55 L224 L223 L222 S54 | L233 L232 L231 S57 L230 L229 L228 S56 | L234 L235 L236 L237 | L238 L239 L240 L241 | L242 L243 L244 L245 | L246 L247 L248 L249 | S58 L250 L251 L252 L253 L254 S59 L255 L256 L257 | S60 L258 L259 L260 S61 L261 L262 L263 | S62 L264 L265 L266 S63 L267 L268 L269 | S64 L270 L271 L272 S65 L273 L274 L275 | L276 L277 S66 L278 L279 L280 L281 L282 S67 L283 | L284 L285 S68 L286 L287 L288 S69 L289 | S70 L290 L291 L292 S71 L293 S72 L294 L295 L296 S73 L297 | L298 L299 S74 L300 L301 L302 S75 L303 | L304 L305 S76 L306 L307 L308 S77 L309 | L310 L311 L312 L313 | S78 L314 L315 L316 S79 L317 L318 L319 | L320 L321 L322 L323
equation "\"d14\" = d10"
equation "\"d18\" = m3 + 0.5 * k"
equation "\"d28\" = m3 + 0.5 * k"
equation "\"m3\" = 3"
equation "\"k\" = 0.4"
body "Solid1"
